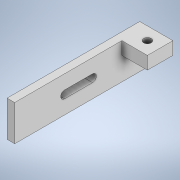
# Autodesk Inventor part: IRSensorMount
Saved by Autodesk Inventor 2020.3 (Build 243373000, 373)
## iProperties
Created: 2020-08-18
Part Number: IRSensorMount
Material: Generic
Document SubType Name: Modeling
Designer: joesp
Density: 1 g/cm^3
Appearance: Default
Author: joesp
Autodesk Inventor part; units mm, degrees
ref_plane "YZ Plane" through (0, 0, 0) normal (1, 0, 0) x (0, 1, 0)
ref_plane "XZ Plane" through (0, 0, 0) normal (0, 1, 0) x (-1, 0, 0)
ref_plane "XY Plane" through (0, 0, 0) normal (0, 0, 1) x (1, 0, 0)
sketch "Sketch2" plane through (0, 0, 0) normal (1, 0, 0) x (0, 1, 0)
  line L0 (0, 0) -> (14, 0)
  line L1 (14, 0) -> (14, -32)
  line L2 (14, -32) -> (0, -32) construction
  line L3 (0, -32) -> (0, 0)
  circle A0 centre (7, -25) radius 1.5
  line L4 (14, -32) -> (14, -52)
  line L5 (14, -52) -> (0, -52)
  line L6 (0, -52) -> (0, -32)
  line L7 (7, -19.5) -> (7, -30.5) construction
  line L8 (5.5, -19.5) -> (5.5, -30.5)
  line L9 (8.5, -30.5) -> (8.5, -19.5)
  arc A1 (8.5, -19.5) -> (5.5, -19.5) centre (7, -19.5) ccw
  arc A2 (5.5, -30.5) -> (8.5, -30.5) centre (7, -30.5) ccw
  point P0 (7, -32)
  dimension "d5" = 32
  dimension "d6" = 14
  dimension "d7" = 3
  dimension "d8" = 7
  dimension "d11" = 20
  constraints: 22 end point, 6 tangent, 4 point on circle, 3 centre point, 3 parallel, 3 perpendicular, 2 midpoint, 2 vertical, 1 horizontal, 1 vertical alignment
  measures "d5" distance of L0.end L1.end
  measures "d6" distance of L1.end L2.end
  measures "d7" diameter of A0
  measures "d8" distance from line of L2 A0.centre
  measures "d11" distance of L1.end L4.end
extrude "Extrusion1" add sketch "Sketch2" along normal blind 3
sketch "Sketch3" plane through (3, 0, 0) normal (1, 0, 0) x (0, 0, -1)
  line L0 (52, 14) -> (42, 14)
  line L1 (42, 14) -> (42, 9)
  line L2 (42, 9) -> (52, 9)
  line L3 (52, 9) -> (52, 14)
  line L4 (52, 0) -> (52, 14) projected
  line L5 (52, 14) -> (0, 14) projected
  dimension "d12" = 5
  dimension "d13" = 10
  constraints: 8 end point, 2 perpendicular, 2 point on line, 1 collinear, 1 parallel
  measures "d12" distance of L0.end L1.end
  measures "d13" distance of L1.end L2.end
extrude "Extrusion2" add sketch "Sketch3" along normal blind 10
sketch "Sketch4" plane through (3, 9, -42) normal (0, -1, 0) x (1, 0, 0)
  circle A0 centre (5, -5) radius 1.5
  line L0 (10, 0) -> (10, -10) projected
  point P0 (-3, 42)
  point P1 (10, -5)
  dimension "d16" = 3
  dimension "d17" = 5
  constraints: 1 centre point, 1 horizontal alignment, 1 midpoint
  measures "d16" diameter of A0
  measures "d17" distance from line of L0 A0.centre
extrude "Extrusion3" cut sketch "Sketch4" against normal through all
body "Solid1"
